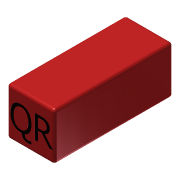
# Autodesk Inventor part: Container 2 2 5 colored color 4
Saved by Autodesk Inventor 2015 (Build 190159000, 159)
## iProperties
Created: 2015-03-07
Part Number: Container 2 2 5 colored color 4
Material: Generic
Document SubType Name: Modeling
Designer: Vukica
Density: 1 g/cm^3
Appearance: Light Red
Author: Vukica
Autodesk Inventor part; units mm, degrees
ref_plane "YZ Plane" through (0, 0, 0) normal (1, 0, 0) x (0, 1, 0)
ref_plane "XZ Plane" through (0, 0, 0) normal (0, 1, 0) x (-1, 0, 0)
ref_plane "XY Plane" through (0, 0, 0) normal (0, 0, 1) x (1, 0, 0)
sketch "Sketch1" plane through (0, 0, 0) normal (0, 0, 1) x (1, 0, 0)
  line L0 (0, 0) -> (50.8, 0)
  line L1 (50.8, 0) -> (50.8, 50.8)
  line L2 (50.8, 50.8) -> (0, 50.8)
  line L3 (0, 50.8) -> (0, 0)
  dimension "d0" = 50.8
  dimension "d1" = 50.8
  constraints: 8 end point, 2 parallel, 1 horizontal, 1 perpendicular
  measures "d0" distance of L1.end L2.end
  measures "d1" distance of L2.end L0.start
extrude "Extrusion1" add sketch "Sketch1" along normal blind 127
sketch "Sketch2" plane through (0, 0, 127) normal (0, 0, 1) x (1, 0, 0)
  line L0 (2.6405, 38.7676) -> (49.0357, 38.7676) construction
  line L1 (49.0357, 38.7676) -> (49.0357, 6.1428) construction
  line L2 (49.0357, 6.1428) -> (2.6405, 6.1428) construction
  line L3 (2.6405, 6.1428) -> (2.6405, 38.7676) construction
  spline S0 degree 2 poles (26.3115, 6.6162) (25.3853, 6.3898) (23.3681, 6.1428) (22.3595, 6.1428) knots 0 0 0 1 2 2 2
  spline S1 degree 2 poles (22.3595, 6.1428) (19.4984, 6.1428) (15.9375, 9.3332) (15.7728, 12.2972) knots 0 0 0 1 2 2 2
  spline S2 degree 2 poles (15.7728, 12.2972) (15.5464, 12.2972) (15.1553, 12.2972) (14.9906, 12.2972) knots 0 0 0 1 2 2 2
  spline S3 degree 2 poles (14.9906, 12.2972) (12.4177, 12.2972) (8.2804, 14.0468) (6.7984, 15.7553) knots 0 0 0 1 2 2 2
  spline S4 degree 2 poles (6.7984, 15.7553) (5.337, 17.4431) (3.7726, 22.3831) (3.7726, 25.5118) knots 0 0 0 1 2 2 2
  spline S5 degree 2 poles (3.7726, 25.5118) (3.7726, 28.7228) (5.3576, 33.5805) (6.819, 35.3096) knots 0 0 0 1 2 2 2
  spline S6 degree 2 poles (6.819, 35.3096) (8.301, 37.018) (12.4383, 38.7676) (14.9906, 38.7676) knots 0 0 0 1 2 2 2
  spline S7 degree 2 poles (14.9906, 38.7676) (17.5841, 38.7676) (21.742, 36.9562) (23.1828, 35.3096) knots 0 0 0 1 2 2 2
  spline S8 degree 2 poles (23.1828, 35.3096) (24.6237, 33.6423) (26.2292, 28.6817) (26.2292, 25.5118) knots 0 0 0 1 2 2 2
  spline S9 degree 2 poles (26.2292, 25.5118) (26.2292, 20.5718) (22.3801, 14.1497) (19.025, 13.0177) knots 0 0 0 1 2 2 2
  spline S10 degree 2 poles (19.025, 13.0177) (19.1073, 12.0708) (19.6013, 10.5476) (19.9924, 10.1154) knots 0 0 0 1 2 2 2
  spline S11 degree 2 poles (19.9924, 10.1154) (20.4658, 9.5802) (21.7626, 9.0862) (22.9153, 9.0862) knots 0 0 0 1 2 2 2
  spline S12 degree 2 poles (22.9153, 9.0862) (23.5945, 9.0862) (25.447, 9.5185) (25.8587, 9.6831) knots 0 0 0 1 2 2 2
  line L4 (25.8587, 9.6831) -> (26.3115, 9.6831)
  line L5 (26.3115, 9.6831) -> (26.3115, 6.6162)
  spline S13 degree 2 poles (22.7094, 25.5118) (22.7094, 28.0436) (21.6185, 31.9339) (20.6305, 33.21) knots 0 0 0 1 2 2 2
  spline S14 degree 2 poles (20.6305, 33.21) (19.6219, 34.5274) (16.7814, 35.8447) (15.0112, 35.8447) knots 0 0 0 1 2 2 2
  spline S15 degree 2 poles (15.0112, 35.8447) (13.1793, 35.8447) (10.4211, 34.5685) (9.3713, 33.21) knots 0 0 0 1 2 2 2
  spline S16 degree 2 poles (9.3713, 33.21) (8.3627, 31.9133) (7.2924, 27.9818) (7.2924, 25.5118) knots 0 0 0 1 2 2 2
  spline S17 degree 2 poles (7.2924, 25.5118) (7.2924, 20.51) (11.4914, 15.1789) (15.0112, 15.1789) knots 0 0 0 1 2 2 2
  spline S18 degree 2 poles (15.0112, 15.1789) (18.531, 15.1789) (22.7094, 20.51) (22.7094, 25.5118) knots 0 0 0 1 2 2 2
  line L6 (49.5914, 12.8324) -> (45.2072, 12.8324)
  line L7 (45.2072, 12.8324) -> (37.1796, 22.9389)
  line L8 (37.1796, 22.9389) -> (33.3099, 22.9389)
  line L9 (33.3099, 22.9389) -> (33.3099, 12.8324)
  line L10 (33.3099, 12.8324) -> (29.9342, 12.8324)
  line L11 (29.9342, 12.8324) -> (29.9342, 38.2324)
  line L12 (29.9342, 38.2324) -> (36.4798, 38.2324)
  spline S19 degree 2 poles (36.4798, 38.2324) (38.6616, 38.2324) (41.605, 37.759) (42.943, 36.8945) knots 0 0 0 1 2 2 2
  spline S20 degree 2 poles (42.943, 36.8945) (44.2809, 36.03) (45.8247, 33.3335) (45.8247, 31.3369) knots 0 0 0 1 2 2 2
  spline S21 degree 2 poles (45.8247, 31.3369) (45.8247, 28.5582) (42.9841, 24.7914) (40.5553, 23.8857) knots 0 0 0 1 2 2 2
  line L13 (40.5553, 23.8857) -> (49.5914, 12.8324)
  spline S22 degree 2 poles (42.3049, 31.0694) (42.3049, 32.1809) (41.5227, 33.8893) (40.6994, 34.445) knots 0 0 0 1 2 2 2
  spline S23 degree 2 poles (40.6994, 34.445) (39.979, 34.9185) (38.0647, 35.3096) (36.665, 35.3096) knots 0 0 0 1 2 2 2
  line L14 (36.665, 35.3096) -> (33.3099, 35.3096)
  line L15 (33.3099, 35.3096) -> (33.3099, 25.7588)
  line L16 (33.3099, 25.7588) -> (36.2739, 25.7588)
  spline S24 degree 2 poles (36.2739, 25.7588) (37.7354, 25.7588) (40.0613, 26.2734) (40.864, 27.0762) knots 0 0 0 1 2 2 2
  spline S25 degree 2 poles (40.864, 27.0762) (41.605, 27.776) (42.3049, 29.752) (42.3049, 31.0694) knots 0 0 0 1 2 2 2
  point P0 (0, 0)
  constraints: 2 other
fillet "Fillet1" radius 3.175 4 edges at (50.8, 50.8, 63.5) (0, 50.8, 63.5) (0, 0, 63.5) (50.8, 0, 63.5)
fillet "Fillet2" radius 3.175 16 edges at (49.8701, 0.9299, 127) (50.8, 25.4, 127) (49.8701, 49.8701, 127) (25.4, 50.8, 127) (0.9299, 49.8701, 127) (0, 25.4, 127) (0.9299, 0.9299, 127) (25.4, 0, 127) (49.8701, 0.9299, 0) (50.8, 25.4, 0) (49.8701, 49.8701, 0) (25.4, 50.8, 0) (0.9299, 49.8701, 0) (0, 25.4, 0) (0.9299, 0.9299, 0) (25.4, 0, 0)
extrude "Extrusion3" cut sketch "Sketch2" against normal blind 0.254
body "Solid1"
